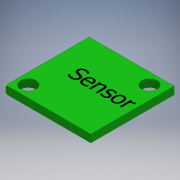
# Autodesk Inventor part: Color
Saved by Autodesk Inventor 2018 (Build 220112000, 112)
## iProperties
Created: 2018-08-18
Part Number: Color
Material: 一般
Document SubType Name: Modeling
Designer: shun2
Density: 1 g/cm^3
Appearance: 濃い緑
Author: shun2
Autodesk Inventor part; units mm, degrees
ref_plane "YZ Plane" through (0, 0, 0) normal (1, 0, 0) x (0, 1, 0)
ref_plane "XZ Plane" through (0, 0, 0) normal (0, 1, 0) x (-1, 0, 0)
ref_plane "XY Plane" through (0, 0, 0) normal (0, 0, 1) x (1, 0, 0)
sketch "スケッチ1" plane through (0, 0, 0) normal (0, 0, 1) x (1, 0, 0)
  line L0 (0, 0) -> (17.8, 0)
  line L1 (17.8, 0) -> (17.76, 17.45)
  line L2 (17.76, 17.45) -> (0, 17.45)
  line L3 (0, 17.45) -> (0, 0)
  line L4 (17.399, 4.007) -> (5.399, 4.007)
  arc A0 (5.399, 4.0388) -> (5.399, 3.9753) centre (5.399, 4.007) ccw
  arc A1 (17.399, 3.9753) -> (17.399, 4.0388) centre (17.399, 4.007) ccw
  line L5 (5.399, 4.007) -> (5.399, 0.507)
  arc A2 (5.3673, 0.507) -> (5.4307, 0.507) centre (5.399, 0.507) ccw
  arc A3 (5.4307, 4.007) -> (5.3673, 4.007) centre (5.399, 4.007) ccw
  line L6 (5.399, 0.507) -> (17.399, 0.507)
  arc A4 (17.399, 0.4753) -> (17.399, 0.5388) centre (17.399, 0.5071) ccw
  arc A5 (5.399, 0.5388) -> (5.399, 0.4753) centre (5.399, 0.5071) ccw
  line L7 (17.399, 0.507) -> (17.399, 4.007)
  arc A6 (17.4307, 4.007) -> (17.3673, 4.007) centre (17.399, 4.007) ccw
  arc A7 (17.3673, 0.507) -> (17.4307, 0.507) centre (17.399, 0.507) ccw
  arc A8 (6.899, 2.8995) -> (6.899, 2.3745) centre (6.899, 2.637) ccw
  arc A9 (6.899, 2.3745) -> (6.899, 2.8995) centre (6.899, 2.637) ccw
  arc A10 (6.899, 2.8995) -> (6.899, 2.3745) centre (6.899, 2.637) ccw
  arc A11 (6.899, 2.3745) -> (6.899, 2.8995) centre (6.899, 2.637) ccw
  arc A12 (8.399, 2.8995) -> (8.399, 2.3745) centre (8.399, 2.637) ccw
  arc A13 (8.399, 2.3745) -> (8.399, 2.8995) centre (8.399, 2.637) ccw
  arc A14 (8.399, 2.8995) -> (8.399, 2.3745) centre (8.399, 2.637) ccw
  arc A15 (8.399, 2.3745) -> (8.399, 2.8995) centre (8.399, 2.637) ccw
  arc A16 (9.899, 2.8995) -> (9.899, 2.3745) centre (9.899, 2.637) ccw
  arc A17 (9.899, 2.3745) -> (9.899, 2.8995) centre (9.899, 2.637) ccw
  arc A18 (9.899, 2.8995) -> (9.899, 2.3745) centre (9.899, 2.637) ccw
  arc A19 (9.899, 2.3745) -> (9.899, 2.8995) centre (9.899, 2.637) ccw
  arc A20 (11.399, 2.8995) -> (11.399, 2.3745) centre (11.399, 2.637) ccw
  arc A21 (11.399, 2.3745) -> (11.399, 2.8995) centre (11.399, 2.637) ccw
  arc A22 (11.399, 2.8995) -> (11.399, 2.3745) centre (11.399, 2.637) ccw
  arc A23 (11.399, 2.3745) -> (11.399, 2.8995) centre (11.399, 2.637) ccw
  arc A24 (12.899, 2.8995) -> (12.899, 2.3745) centre (12.899, 2.637) ccw
  arc A25 (12.899, 2.3745) -> (12.899, 2.8995) centre (12.899, 2.637) ccw
  arc A26 (12.899, 2.8995) -> (12.899, 2.3745) centre (12.899, 2.637) ccw
  arc A27 (12.899, 2.3745) -> (12.899, 2.8995) centre (12.899, 2.637) ccw
  arc A28 (14.399, 2.8995) -> (14.399, 2.3745) centre (14.399, 2.637) ccw
  arc A29 (14.399, 2.3745) -> (14.399, 2.8995) centre (14.399, 2.637) ccw
  arc A30 (14.399, 2.8995) -> (14.399, 2.3745) centre (14.399, 2.637) ccw
  arc A31 (14.399, 2.3745) -> (14.399, 2.8995) centre (14.399, 2.637) ccw
  arc A32 (15.899, 2.8995) -> (15.899, 2.3745) centre (15.899, 2.637) ccw
  arc A33 (15.899, 2.3745) -> (15.899, 2.8995) centre (15.899, 2.637) ccw
  arc A34 (15.899, 2.8995) -> (15.899, 2.3745) centre (15.899, 2.637) ccw
  arc A35 (15.899, 2.3745) -> (15.899, 2.8995) centre (15.899, 2.637) ccw
  line L8 (0, 17.45) -> (17.8, 17.45)
  line L9 (17.8, 17.45) -> (17.8, 0)
  line L10 (17.8, 0) -> (0, 0)
  line L11 (0, 0) -> (0, 17.45)
  circle A36 centre (15.0106, 15.0866) radius 1.6
  circle A37 centre (2.3106, 2.3866) radius 1.6
  dimension "d0" = 3.2
  dimension "d1" = 3.2
  dimension "d2" = 12.7
  dimension "d3" = 12.7
  constraints: 72 point on circle, 38 centre point, 24 end point, 2 parallel, 1 horizontal, 1 perpendicular
  measures "d0" diameter of A36
  measures "d1" diameter of A37
  measures "d2" horizontal distance of A36.centre A37.centre
  measures "d3" horizontal distance of A37.centre A36.centre
extrude "押し出し1" add sketch "スケッチ1" along normal blind 1.6 contours L3 L2 L1 L0 | L1 L8 L9 | L7 L6 L5 L4 | L4 A6 A1 L7 | L4 L5 A0 A3 | A4 A7 L6 L7 | L5 L6 A2 A5 | A9 A8 | A13 A12 | A17 A16 | A21 A20 | A25 A24 | A29 A28 | A33 A32
sketch "スケッチ2" plane through (0, 0, 1.6) normal (0, 0, 1) x (1, 0, 0)
  line L0 (4.476, 11.19) -> (11.1005, 11.19) construction
  line L1 (11.1005, 11.19) -> (11.1005, 8.2657) construction
  line L2 (11.1005, 8.2657) -> (4.476, 8.2657) construction
  line L3 (4.476, 8.2657) -> (4.476, 11.19) construction
  point P0 (0, 0)
  constraints: 2 other
sketch "スケッチ3" plane through (0, 0, 0) normal (0, 0, -1) x (-1, 0, 0)
  line L0 (-15.9942, 10.8916) -> (2.8001, 10.8916) construction
  line L1 (2.8001, 10.8916) -> (2.8001, 7.6653) construction
  line L2 (2.8001, 7.6653) -> (-15.9942, 7.6653) construction
  line L3 (-15.9942, 7.6653) -> (-15.9942, 10.8916) construction
  line L4 (-17.4862, 3.551) -> (-6.147, 3.551)
  line L5 (-6.147, 3.551) -> (-6.147, 0.3282)
  line L6 (-6.147, 0.3282) -> (-17.4862, 0.3282)
  line L7 (-17.4862, 0.3282) -> (-17.4862, 3.551)
  point P0 (0, 0)
  constraints: 8 end point, 2 parallel, 1 horizontal, 1 perpendicular, 2 other
